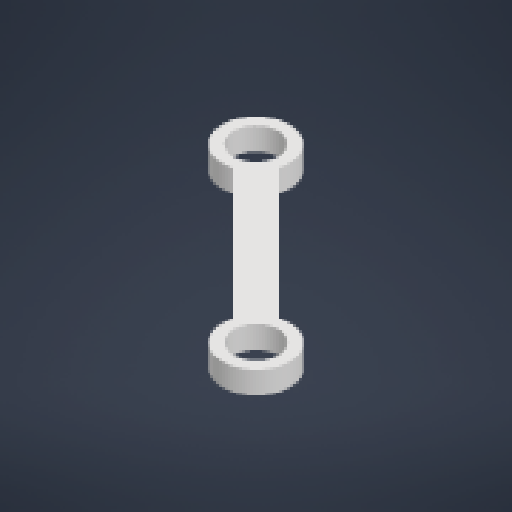
# Autodesk Inventor part: Pillar_corner_v2
Saved by Autodesk Inventor 2026 (Build 300175050, 175E)
## iProperties
Created: 2026-06-21
Part Number: Pillar_corner_v2
Material: Generic
Document SubType Name: Modeling
Designer: sniel
Density: 1 g/cm^3
Appearance: Default
Author: sniel
Autodesk Inventor part; units mm, degrees
ref_plane "YZ Plane" through (0, 0, 0) normal (1, 0, 0) x (0, 1, 0)
ref_plane "XZ Plane" through (0, 0, 0) normal (0, 1, 0) x (-1, 0, 0)
ref_plane "XY Plane" through (0, 0, 0) normal (0, 0, 1) x (1, 0, 0)
sketch "Sketch1" plane through (0, 0, 0) normal (0, 1, 0) x (-1, 0, 0)
  circle A0 centre (-0.0502, 38.3312) radius 4.925
  line L0 (-0.0502, 38.3312) -> (0, 0)
  circle A1 centre (38.3312, 0.0502) radius 4.925
  line L1 (38.3312, 0.0502) -> (0, 0)
  circle A2 centre (38.3312, 0.0502) radius 5
  circle A3 centre (-0.0502, 38.3312) radius 5
  circle A4 centre (-0.0502, 38.3312) radius 7.5
  circle A5 centre (38.3312, 0.0502) radius 7.5
  line L2 (38.3312, 0.0502) -> (-0.0502, 38.3312)
  line L3 (21.6405, 21.6907) -> (16.6405, 21.6907)
  line L4 (16.6405, 21.6907) -> (16.6405, 16.6907)
  line L5 (16.6405, 16.6907) -> (21.6405, 16.6907)
  line L6 (21.6405, 16.6907) -> (21.6405, 21.6907)
  line L7 (21.6405, 21.6907) -> (16.6405, 16.6907) construction
  line L8 (16.6405, 21.6907) -> (21.6405, 16.6907) construction
  line L9 (21.6405, 21.6907) -> (2.4716, 40.8596)
  line L10 (21.6405, 21.6907) -> (37.3312, 6)
  line L11 (16.6405, 16.6907) -> (-2.5284, 35.8596)
  line L12 (16.6405, 16.6907) -> (32.3312, 1)
  point P0 (0, 0)
  point P1 (0, 0)
  point P2 (19.1405, 19.1907)
  point P3 (36.1157, 7.2155)
  point P4 (7.1385, 36.1927)
  point P5 (2.1653, 31.1659)
  point P6 (31.1425, 2.1887)
  dimension "d0" = 10
  dimension "d1" = 10
  dimension "d2" = 15
  dimension "d3" = 15
  dimension "d4" = 5
  dimension "d5" = 5
  constraints: 26 end point, 6 centre point, 4 coincident, 3 midpoint, 3 parallel, 2 perpendicular, 1 horizontal
  measures "d0" diameter of A2
  measures "d1" diameter of A3
  measures "d2" diameter of A4
  measures "d3" diameter of A5
  measures "d4" distance of L5.end L4.end
  measures "d5" distance of L4.end L3.end
extrude "Extrusion1" add sketch "Sketch1" along normal blind 5 contours L9 A4 L2 A3 | A3 L0 A4 L9 | L2 A4 L11 A3 | A3 L11 A4 L0 | L9 L3 L4 L2 A4 | L2 L4 L11 A4 | L6 L2 L4 L3 | L10 A5 L2 L6 | L2 L6 L5 L4 | L2 A5 L12 L5 L6 | A5 L1 A2 L2 | A5 L2 A2 L1
body "Solid1"
